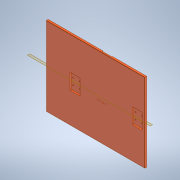
# Autodesk Inventor part: Yplate
Saved by Autodesk Inventor 2020 (Build 240168000, 168)
## iProperties
Created: 2019-06-14
Part Number: Yplate
Material: Phenolic Resin
Document SubType Name: Modeling
Designer: LillaHunden
Density: 1.38 g/cm^3
Appearance: Smooth - Light Orange
Author: LillaHunden
Autodesk Inventor part; units mm, degrees
ref_plane "YZ Plane" through (0, 0, 0) normal (1, 0, 0) x (0, 1, 0)
ref_plane "XZ Plane" through (0, 0, 0) normal (0, 1, 0) x (-1, 0, 0)
ref_plane "XY Plane" through (0, 0, 0) normal (0, 0, 1) x (1, 0, 0)
sketch "Sketch1" plane through (0, 0, 0) normal (0, 0, 1) x (1, 0, 0)
  line L0 (170, 120) -> (-170, 120)
  line L1 (-170, 120) -> (-170, -120)
  line L2 (-170, -120) -> (170, -120)
  line L3 (170, -120) -> (170, 120)
  line L4 (170, 120) -> (-170, -120) construction
  line L5 (-170, 120) -> (170, -120) construction
  point P0 (0, 0)
  dimension "d0" = 340
  dimension "d1" = 240
  constraints: 12 end point, 2 midpoint, 2 parallel, 1 horizontal, 1 perpendicular
  measures "d0" distance of L2.end L1.end
  measures "d1" distance of L1.end L0.end
extrude "Extrusion1" add sketch "Sketch1" along normal blind 6.35
ref_plane "Work Plane1" through (-170, 0, 0) normal (0, 1, 0) x (1, 0, 0)
sketch "Sketch2" plane through (0, 0, 6.35) normal (0, 0, 1) x (1, 0, 0)
  line L0 (161, -16) -> (161, 16) construction
  line L1 (160.5, -21) -> (134.5, -21) construction
  line L2 (134.5, 21) -> (160.5, 21) construction
  line L3 (134, 16) -> (134, -16) construction
  line L4 (-49, -20.074) -> (-55.5, -20.074) construction
  line L5 (-55.5, -20.074) -> (-55.5, 11.926) construction
  line L6 (-55.5, 11.926) -> (-49, 11.926) construction
  line L7 (-49, -20.074) -> (-49, 11.926) construction
  circle A0 centre (-52.5, 5.926) radius 1.35 construction
  circle A1 centre (-52.5, -14.074) radius 1.375 construction
  line L8 (-56, 11.926) -> (-56, -20.074) construction
  line L9 (-29, -20.074) -> (-29, 11.926) construction
  line L10 (-55.5, -26.074) -> (-29.5, -26.074) construction
  line L11 (-29.5, 17.926) -> (-55.5, 17.926) construction
  line L12 (-27, 19.926) -> (-58, 19.926)
  line L13 (-58, 19.926) -> (-58, -28.074)
  line L14 (-58, -28.074) -> (-27, -28.074)
  line L15 (-27, -28.074) -> (-27, 19.926)
  line L16 (132, 24) -> (163, 24)
  line L17 (163, 24) -> (163, -24)
  line L18 (163, -24) -> (132, -24)
  line L19 (132, -24) -> (132, 24)
  point P0 (0, 0)
  point P1 (-42.5, 19.926)
  point P2 (-42.5, 17.926)
  point P3 (147.5, 24)
  point P4 (147.5, 21)
  point P5 (132, 0)
  point P6 (134, 0)
  point P7 (-58, -4.074)
  point P8 (-29, -4.074)
  dimension "d4" = 2
  dimension "d5" = 2
  constraints: 16 end point, 8 midpoint, 6 parallel, 2 horizontal, 2 horizontal alignment, 2 perpendicular, 2 vertical alignment
  measures "d4" distance between parallel lines of L11 L12
  measures "d5" distance between parallel lines of L9 L15
extrude "Extrusion2" cut sketch "Sketch2" against normal blind 4.35
fillet "Fillet1" radius 1.7 8 edges at (-58, 19.926, 4.175) (-27, 19.926, 4.175) (-27, -28.074, 4.175) (-58, -28.074, 4.175) (163, -24, 4.175) (132, -24, 4.175) (132, 24, 4.175) (163, 24, 4.175)
sketch "Sketch3" plane through (0, 0, 0) normal (0, 0, -1) x (-1, 0, 0)
  point P0 (-157.5, 10)
  point P1 (-137.5, 10)
  point P2 (-137.5, -10)
  point P3 (-157.5, -10)
  point P4 (52.5, -14.074)
  point P5 (32.5, -14.074)
  point P6 (32.5, 5.926)
  point P7 (52.5, 5.926)
hole "Hole1" at (157.5, 10, 0) at (137.5, 10, 0) at (137.5, -10, 0) at (157.5, -10, 0) at (-52.5, -14.074, 0) at (-32.5, -14.074, 0) at (-32.5, 5.926, 0) at (-52.5, 5.926, 0) direction (0, 0, 1) diameter 3.4 depth 2 countersink diameter 6.3 countersink angle 90
sketch "Sketch7" plane through (0, 0, 0) normal (0, 0, -1) x (-1, 0, 0)
  line L0 (-38.71, 124) -> (-38.71, 121) construction
  line L1 (-62.71, 121) -> (-62.71, 124) construction
  line L2 (-65.71, 110) -> (-35.71, 110)
  line L3 (-35.71, 110) -> (-35.71, 120)
  line L4 (-35.71, 120) -> (-65.71, 120)
  line L5 (-65.71, 120) -> (-65.71, 110)
  line L6 (-170, 120) -> (170, 120) projected
  point P0 (0, 0)
  point P1 (-57.5175, 113)
  point P2 (-50.71, 120)
  dimension "d35" = 3
  dimension "d36" = 3
  dimension "d37" = 3
  constraints: 8 end point, 2 parallel, 1 horizontal, 1 midpoint, 1 perpendicular, 1 point on line, 1 other
  measures "d35" distance from line of L2 point (-57.518, 113)
  measures "d36" distance between parallel lines of L1 L5
  measures "d37" distance between parallel lines of L3 L0
extrude "Extrusion4" cut sketch "Sketch7" against normal blind 2.25
fillet "Fillet2" radius 1.7 2 edges at (65.71, 110, 1.125) (35.71, 110, 1.125)
move faces "Move1" translate (40, 0, 0) faces at (-170, 40, 4.2333)
sketch "Sketch8" plane through (0, 0, 0) normal (0, 0, -1) x (-1, 0, 0)
  point P0 (-26.7, -10.4291)
  point P1 (-34.7, -10.4291)
  point P2 (-42.7, -10.4291)
  point P3 (-50.7, -10.4291)
hole "Hole6" at (26.7, -10.4291, 0) at (34.7, -10.4291, 0) at (42.7, -10.4291, 0) at (50.7, -10.4291, 0) direction (0, 0, 1) diameter 3.4 depth 6.35 countersink diameter 6.4 countersink angle 90
chamfer "Chamfer1" distance 0.5 angle 45 9 edges at (170, 0, 6.35) (20, 120, 6.35) (20, -120, 6.35) (-130, 0, 6.35) (20, -120, 0) (-130, 0, 0) (-47.145, 120, 0) (117.855, 120, 0) (170, 0, 0)
equation "\"d37\" = d36"
body "Solid1"
